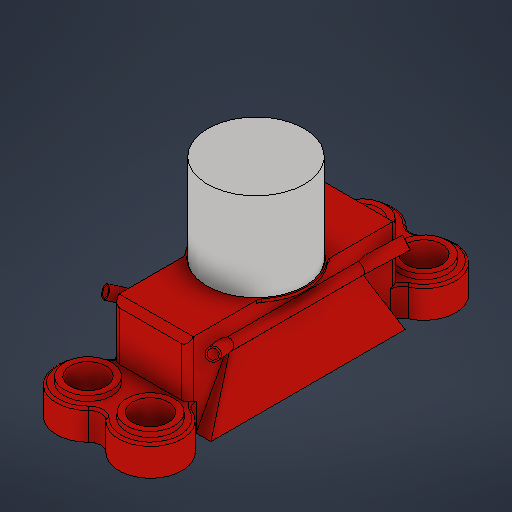
# Autodesk Inventor part: SACMI PH1500 PRESS TOP
Saved by Autodesk Inventor 2025 (Build 290162000, 162)
## iProperties
Created: 2024-05-02
Part Number: SACMI PH1500 PRESS TOP
Material: Generic
Document SubType Name: Modeling
Designer: zulet
Density: 1 g/cm^3
Appearance: Orange-Red
Author: zulet
Autodesk Inventor part; units mm, degrees
ref_plane "YZ Plane" through (0, 0, 0) normal (1, 0, 0) x (0, 1, 0)
sketch "Sketch1" plane through (0, 0, 0) normal (0, 1, 0) x (-1, 0, 0)
  line L0 (250, -750) -> (-250, -750)
  line L1 (-250, -750) -> (-250, 750)
  line L2 (-250, 750) -> (250, 750)
  line L3 (250, 750) -> (250, -750)
  line L4 (250, -750) -> (-250, 750) construction
  line L5 (-250, -750) -> (250, 750) construction
  circle A0 centre (210, 920) radius 120
  line L6 (0, 750) -> (0, -750) construction
  line L7 (250, 0) -> (-250, 0) construction
  circle A1 centre (210, 920) radius 212.5
  circle A2 centre (-210, 920) radius 120
  circle A3 centre (-210, 920) radius 212.5
  circle A4 centre (210, -920) radius 120
  circle A5 centre (210, -920) radius 212.5
  circle A6 centre (-210, -920) radius 212.5
  circle A7 centre (-210, -920) radius 120
  point P0 (0, 0)
  point P1 (-250, 711.2987)
  point P2 (-250, -711.2987)
  point P3 (0, -952.5)
  point P4 (250, -711.2987)
  point P5 (250, 711.2987)
  point P6 (0, 952.5)
  dimension "d0" = 500
  dimension "d1" = 1500
  dimension "d2" = 240
  dimension "d3" = 210
  dimension "d4" = 920
  dimension "d5" = 425
  constraints: 16 end point, 8 centre point, 6 midpoint, 6 symmetric about line, 4 coincident, 2 parallel, 1 horizontal, 1 perpendicular, 6 other
  measures "d0" distance of L1.end L2.end
  measures "d1" distance of L0.end L1.end
  measures "d2" diameter of A0
  measures "d3" distance from line of A0.centre L6
  measures "d4" distance from line of L7 A0.centre
  measures "d5" diameter of A1
extrude "Extrusion1" add sketch "Sketch1" along normal blind 200
sketch "Sketch2" plane through (0, 200, 0) normal (0, 1, 0) x (1, 0, 0)
  line L0 (-250, 711.2987) -> (-250, -711.2987) projected
  line L1 (250, 711.2987) -> (-250, 711.2987)
  line L2 (-250, 711.2987) -> (-250, -711.2987)
  line L3 (-250, -711.2987) -> (250, -711.2987)
  line L4 (250, -711.2987) -> (250, 711.2987)
  line L5 (250, 711.2987) -> (-250, -711.2987) construction
  line L6 (-250, 711.2987) -> (250, -711.2987) construction
  point P0 (0, 0)
  point P1 (-250, 711.2987)
  constraints: 12 end point, 2 midpoint, 2 parallel, 1 horizontal, 1 perpendicular
extrude "Extrusion2" add sketch "Sketch2" along normal blind 370
sketch "Sketch3" plane through (0, 570, 0) normal (0, 1, 0) x (1, 0, 0)
  circle A0 centre (0, 0) radius 325
  dimension "d10" = 650
  constraints: 1 centre point, 1 coincident
  measures "d10" diameter of A0
extrude "Extrusion3" add sketch "Sketch3" along normal blind 590
fillet "Fillet1" radius 80 6 edges at (250, 100, 711.2987) (250, 100, -711.2987) (0, 100, 952.5) (0, 100, -952.5) (-250, 100, -711.2987) (-250, 100, 711.2987)
chamfer "Chamfer1" distance 40 angle 45 2 edges at (0, 570, 711.2987) (0, 570, -711.2987)
sketch "Sketch4" plane through (0, 200, 0) normal (0, 1, 0) x (1, 0, 0)
  circle A0 centre (-210, -920) radius 120 projected
  circle A1 centre (210, -920) radius 120 projected
  circle A2 centre (-210, 920) radius 120 projected
  circle A3 centre (210, 920) radius 120 projected
  circle A4 centre (-210, -920) radius 160
  circle A5 centre (210, -920) radius 160
  circle A6 centre (-210, 920) radius 160
  circle A7 centre (210, 920) radius 160
  point P0 (0, 0)
  dimension "d17" = 40
  dimension "d18" = 40
  dimension "d19" = 40
  dimension "d20" = 40
  constraints: 4 centre point
  measures "d17" radial gap between concentric circles of A0 A4
  measures "d18" radial gap between concentric circles of A1 A5
  measures "d19" radial gap between concentric circles of A2 A6
  measures "d20" radial gap between concentric circles of A3 A7
extrude "Extrusion4" add sketch "Sketch4" along normal blind 35
fillet "Fillet2" radius 15 10 edges at (0, 200, 1043.6081) (383.9566, 200, 1042.0465) (262.8225, 200, 696.6904) (-262.8225, 200, 696.6904) (-383.9566, 200, 1042.0465) (0, 200, -1043.6081) (-383.9566, 200, -1042.0465) (-262.8225, 200, -696.6904) (262.8225, 200, -696.6904) (383.9566, 200, -1042.0465)
sketch "Sketch5" plane through (250, 570, 207.6656) normal (1, 0, 0) x (0, 0, -1)
  line L0 (-445.5831, -570) -> (860.9143, -570) projected
  line L1 (-445.5831, -570) -> (-242.3344, -190)
  line L2 (-242.3344, -190) -> (657.6656, -190)
  line L3 (657.6656, -190) -> (860.9143, -570)
  line L4 (207.6656, -190) -> (207.6656, -570) construction
  dimension "d26" = 380
  dimension "d27" = 900
  constraints: 8 end point, 1 midpoint, 1 parallel, 1 perpendicular
  measures "d26" distance between parallel lines of L0 L2
  measures "d27" distance of L1.end L2.end
extrude "Extrusion5" add sketch "Sketch5" along normal blind 100
chamfer "Chamfer2" distance 380 distance2 80 1 edges at (350, 380, 0) measured on face at (350, 379.5, 0)
ref_plane "Work Plane1" through (250, 380, 450) normal (0, 0, 1) x (1, 0, 0)
sketch "Sketch6" plane through (250, 380, 450) normal (0, 0, 1) x (1, 0, 0)
  line L0 (0, 0) -> (20, 0) projected
  circle A0 centre (0, 34.641) radius 40
  circle A1 centre (0, 34.641) radius 30
  line L1 (0, -180) -> (0, 150) projected
  point P0 (-250, -380)
  point P1 (0, 74.641)
  point P2 (0, 64.641)
  point P3 (0, 4.641)
  dimension "d35" = 80
  dimension "d34" = 60
  constraints: 1 centre point, 1 coincident, 1 point on line, 3 other
  measures "d34" diameter of A1
extrude "Extrusion6" add sketch "Sketch6" against normal up to surface (900 mm away) contours L1 A1 A0 L0
sketch "Sketch8" plane through (250, 380, 450) normal (0, 0, 1) x (1, 0, 0)
  arc A0 (0, 4.641) -> (0, 64.641) centre (0, 34.641) ccw projected
  circle A1 centre (0, 34.641) radius 30
  arc A2 (20, 0) -> (0, 74.641) centre (0, 34.641) ccw projected
  circle A3 centre (0, 34.641) radius 40
  point P0 (-250, -380)
  constraints: 2 coincident, 2 vertical alignment, 4 other
sketch3d "3D Sketch1"
ref_plane "Work Plane2" through (361.8034, 414.641, 650) normal (0.8728716, 0, -0.48795) x (0, 1, 0)
sketch "Sketch9" plane through (361.8034, 414.641, 650) normal (0.8728716, 0, -0.48795) x (0, 1, 0)
  line L0 (72.5045, 12) -> (-47.4955, -262.9545)
  line L1 (-47.4955, -262.9545) -> (-56.6606, -258.9545)
  line L2 (-56.6606, -258.9545) -> (63.3394, 16)
  line L3 (63.3394, 16) -> (72.5045, 12)
  line L4 (0, -229.1288) -> (100, 0) projected
  line L5 (100, 0) -> (72.5045, 12) construction
  point P0 (-414.641, -743.9085)
  dimension "d41" = 30
  dimension "d42" = 10
  dimension "d43" = 300
  constraints: 10 end point, 3 parallel, 2 perpendicular
  measures "d41" distance of L4.end L0.start
  measures "d42" distance of L2.end L0.start
  measures "d43" distance of L1.end L2.end
revolve "Revolution1" add sketch "Sketch9" angle 360 about axis through (250, 414.641, 450) along (0.4472136, 0.4, 0.8)
mirror "Mirror1" about plane through (0, 0, 0) normal (0, 0, 1) of "Revolution1"
mirror "Mirror2" about plane through (0, 0, 0) normal (1, 0, 0) of "Extrusion5", "Extrusion6", "Revolution1", "Mirror1"
fillet "Fillet5" radius 40 4 edges at (250, 365, 711.2987) (-250, 365, 711.2987) (250, 365, -711.2987) (-250, 365, -711.2987)
sketch "Sketch10" plane through (0, 570, 0) normal (0, -1, 0) x (1, 0, 0)
  line L0 (250, 207.6656) -> (250, -207.6656) construction
  arc A0 (250, -207.6656) -> (250, 207.6656) centre (0, 0) ccw construction
  line L1 (-250, -207.6656) -> (-250, 207.6656) construction
  arc A1 (-250, 207.6656) -> (-250, -207.6656) centre (0, 0) ccw construction
  line L2 (235, -245.7132) -> (235, 245.7132)
  arc A2 (235, -245.7132) -> (235, 245.7132) centre (0, 0) ccw
  line L3 (-235, 245.7132) -> (-235, -245.7132)
  arc A3 (-235, 245.7132) -> (-235, -245.7132) centre (0, 0) ccw
  dimension "d46" = 15
  dimension "d47" = 15
  constraints: 4 end point, 4 point on circle, 2 centre point, 2 other
  measures "d46" distance between parallel lines of L0 L2
  measures "d47" radial gap between concentric circles of A1 A3
extrude "Extrusion7" add sketch "Sketch10" along normal blind 20
fillet "Fillet6" radius 40 4 edges at (-250, 560, -230.4344) (-250, 560, 230.4344) (250, 560, 230.4344) (250, 560, -230.4344)
sketch "Sketch11" plane through (0, 570, 0) normal (0, 1, 0) x (1, 0, 0)
  circle A0 centre (0, 0) radius 325 projected
  circle A1 centre (0, 0) radius 330
  dimension "d51" = 5
  constraints: 1 centre point
  measures "d51" radial gap between concentric circles of A0 A1
extrude "Extrusion8" cut sketch "Sketch11" against normal blind 10
sketch "Sketch12" plane through (0, 550, 0) normal (0, -1, 0) x (1, 0, 0)
  arc A0 (-259.4737, 219.7121) -> (-259.4737, -219.7121) centre (0, 0) ccw projected
  line L0 (-250, 245.5606) -> (-250, -245.5606) projected
  line L1 (-250, 0) -> (-340, 0) construction
  circle A1 centre (-315, 0) radius 7.5
  circle A2 centre (-309.9378, -56.2454) radius 7.5
  circle A3 centre (-294.914, -110.6831) radius 7.5
  circle A4 centre (-270.4114, -161.5633) radius 7.5
  circle A5 centre (-237.2175, -207.2507) radius 7.5
  circle A6 centre (-196.3993, -246.2769) radius 7.5
  circle A7 centre (-149.2686, -277.3876) radius 7.5
  circle A8 centre (-97.3404, -299.5828) radius 7.5
  circle A9 centre (-42.2835, -312.1492) radius 7.5
  circle A10 centre (14.1324, -314.6828) radius 7.5
  circle A11 centre (70.0941, -307.1023) radius 7.5
  circle A12 centre (123.8029, -289.6512) radius 7.5
  circle A13 centre (173.5325, -262.8906) radius 7.5
  circle A14 centre (217.6847, -227.6804) radius 7.5
  circle A15 centre (254.8404, -185.1524) radius 7.5
  circle A16 centre (283.8052, -136.6734) radius 7.5
  circle A17 centre (303.6483, -83.8016) radius 7.5
  circle A18 centre (313.7319, -28.2364) radius 7.5
  circle A19 centre (313.7319, 28.2364) radius 7.5
  circle A20 centre (303.6483, 83.8016) radius 7.5
  circle A21 centre (283.8052, 136.6734) radius 7.5
  circle A22 centre (254.8404, 185.1524) radius 7.5
  circle A23 centre (217.6847, 227.6804) radius 7.5
  circle A24 centre (173.5325, 262.8906) radius 7.5
  circle A25 centre (123.8029, 289.6512) radius 7.5
  circle A26 centre (70.0941, 307.1023) radius 7.5
  circle A27 centre (14.1324, 314.6828) radius 7.5
  circle A28 centre (-42.2835, 312.1492) radius 7.5
  circle A29 centre (-97.3404, 299.5828) radius 7.5
  circle A30 centre (-149.2686, 277.3876) radius 7.5
  circle A31 centre (-196.3993, 246.2769) radius 7.5
  circle A32 centre (-237.2175, 207.2507) radius 7.5
  circle A33 centre (-270.4114, 161.5633) radius 7.5
  circle A34 centre (-294.914, 110.6831) radius 7.5
  circle A35 centre (-309.9378, 56.2454) radius 7.5
  dimension "d54" = 15
  dimension "d55" = 65
  dimension "d58" = 360
  constraints: 35 centre point, 2 end point, 1 midpoint, 1 point on circle, 1 point on line, 71 other
  measures "d54" diameter of A1
  measures "d55" distance from line of L0 A1.centre
extrude "Extrusion9" add sketch "Sketch12" along normal blind 10 contours A1 | A2 | A3 | A4 | A15 | A16 | A17 | A18 | A19 | A20 | A21 | A22 | A33 | A34 | A35
sketch "Sketch13" plane through (0, 0, 0) normal (0, -1, 0) x (1, 0, 0)
  line L0 (200, 500) -> (-200, 500) construction
  line L1 (-200, 500) -> (-200, -500) construction
  line L2 (-200, -500) -> (200, -500) construction
  line L3 (200, -500) -> (200, 500) construction
  line L4 (200, 500) -> (-200, -500) construction
  line L5 (-200, 500) -> (200, -500) construction
  circle A0 centre (-200, -500) radius 30
  circle A1 centre (-200, -250) radius 30
  circle A2 centre (-200, 0) radius 30
  circle A3 centre (-200, 250) radius 30
  circle A4 centre (-200, 500) radius 30
  circle A5 centre (200, -500) radius 30
  circle A6 centre (200, -250) radius 30
  circle A7 centre (200, 0) radius 30
  circle A8 centre (200, 250) radius 30
  circle A9 centre (200, 500) radius 30
  point P0 (0, 0)
  dimension "d62" = 400
  dimension "d63" = 1000
  dimension "d64" = 60
  dimension "d67" = 250
  dimension "d70" = 400
  constraints: 12 end point, 10 centre point, 2 horizontal, 2 midpoint, 2 parallel, 1 coincident, 1 perpendicular, 1 vertical, 18 other
  measures "d62" distance of L2.end L1.end
  measures "d63" distance of L1.end L0.end
  measures "d64" diameter of A0
  measures "d67" distance of A0.centre A1.centre
  measures "d70" distance of A0.centre A5.centre
extrude "Extrusion10" cut sketch "Sketch13" against normal blind 20
equation "\"d18\" = d17"
equation "\"d19\" = d17"
equation "\"d20\" = d17"
equation "\"d67\" = 0.25 * d63"
equation "\"d70\" = d62"
body "Solid1"
